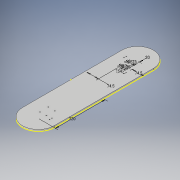
# Autodesk Inventor part: sfp_smartboard_lower_deck
Saved by Autodesk Inventor 2019 (Build 230136000, 136)
## iProperties
Created: 2019-02-09
Part Number: sfp_smartboard_lower_deck
Material: 一般
Document SubType Name: Modeling
Designer: drago
Density: 1 g/cm^3
Appearance: 既定
Author: drago
Autodesk Inventor part; units mm, degrees
ref_plane "YZ Plane" through (0, 0, 0) normal (1, 0, 0) x (0, 1, 0)
ref_plane "XZ Plane" through (0, 0, 0) normal (0, 1, 0) x (-1, 0, 0)
ref_plane "XY Plane" through (0, 0, 0) normal (0, 0, 1) x (1, 0, 0)
sketch "スケッチ1" plane through (0, 0, 0) normal (0, 1, 0) x (-1, 0, 0)
  point P0 (0, 0)
sketch "スケッチ2" plane through (0, 0, 0) normal (0, 1, 0) x (-1, 0, 0)
  line L0 (0.845, -60.969) -> (0.845, -330.969)
  line L1 (0, 0) -> (0, -1.5537)
  line L2 (-202.155, -60.969) -> (-202.155, -330.969)
  arc A0 (-202.155, -330.969) -> (0.845, -330.969) centre (-100.655, -330.969) ccw
  line L3 (0.845, -60.969) -> (0.845, 309.031)
  line L4 (-202.155, -60.969) -> (-202.155, 309.031)
  arc A1 (0.845, 309.031) -> (-202.155, 309.031) centre (-100.655, 309.031) ccw
  dimension "d0" = 270
  dimension "d1" = 203
  constraints: 10 end point, 4 point on circle, 3 vertical, 2 centre point, 2 tangent, 1 parallel
  measures "d0" distance of L0.start L0.end
  measures "d1" distance of L0.start L2.start
extrude "押し出し1" add sketch "スケッチ2" against normal blind 10
sketch "スケッチ4" plane through (0, -10, 0) normal (0, -1, 0) x (1, 0, 0)
  line L0 (73.655, -234.969) -> (127.655, -234.969)
  line L1 (127.655, -234.969) -> (127.655, -310.969)
  line L2 (127.655, -310.969) -> (73.655, -310.969)
  line L3 (73.655, -310.969) -> (73.655, -234.969)
  line L4 (202.155, -330.969) -> (202.155, 309.031) projected
  line L5 (-0.845, 309.031) -> (-0.845, -330.969) projected
  arc A0 (-0.845, -330.969) -> (202.155, -330.969) centre (100.655, -330.969) ccw projected
  line L6 (-0.845, -10.969) -> (202.155, -10.969)
  arc A1 (202.155, 309.031) -> (-0.845, 309.031) centre (100.655, 309.031) ccw projected
  line L7 (73.655, 213.031) -> (127.655, 213.031)
  line L8 (127.655, 213.031) -> (127.655, 289.031)
  line L9 (127.655, 289.031) -> (73.655, 289.031)
  line L10 (73.655, 289.031) -> (73.655, 213.031)
  circle A2 centre (79.655, -299.219) radius 2.75
  line L11 (100.655, -256.1001) -> (100.655, -272.969)
  circle A3 centre (79.655, -245.219) radius 2.75
  circle A4 centre (121.655, -299.219) radius 2.75
  circle A5 centre (121.655, -245.219) radius 2.75
  line L12 (73.655, 213.031) -> (127.655, 213.031)
  line L13 (127.655, 213.031) -> (127.655, 289.031)
  line L14 (127.655, 289.031) -> (73.655, 289.031)
  line L15 (73.655, 289.031) -> (73.655, 213.031)
  circle A6 centre (79.655, 277.281) radius 2.75
  line L16 (100.655, 234.1622) -> (100.655, 251.031)
  circle A7 centre (79.655, 223.281) radius 2.75
  circle A8 centre (121.655, 223.281) radius 2.75
  circle A9 centre (121.655, 277.281) radius 2.75
  point P0 (0, 0)
  dimension "d4" = 74.5
  dimension "d5" = 74.5
  dimension "d6" = 54
  dimension "d7" = 76
  dimension "d8" = 20
  dimension "d9" = 320
  dimension "d17" = 5.5
  dimension "d18" = 11.75
  dimension "d19" = 6
  dimension "d20" = 27
  dimension "d21" = 5.5
  dimension "d22" = 10.25
  dimension "d23" = 6
  constraints: 30 end point, 12 symmetric about line, 8 centre point, 2 midpoint, 2 parallel, 2 perpendicular, 1 horizontal, 1 vertical, 6 other
  measures "d4" distance between parallel lines of L4 L1
  measures "d5" distance between parallel lines of L5 L3
  measures "d6" distance of L0.start L0.end
  measures "d7" distance between parallel lines of L2 L0
  measures "d8" distance from line of A0.centre L2
  measures "d9" distance from line of A1.centre L6
  measures "d17" diameter of A2
  measures "d18" distance from line of L2 A2.centre
  measures "d19" distance from line of L3 A2.centre
  measures "d20" distance between parallel lines of L3 L11
  measures "d21" diameter of A3
  measures "d22" distance from line of L0 A3.centre
  measures "d23" distance from line of L3 A3.centre
hole "穴2" at (79.655, -10, -245.219) at (79.655, -10, -299.219) at (121.655, -10, -299.219) at (121.655, -10, -245.219) direction (0, 1, 0) diameter 5.5 end through all
hole "穴3" at (79.655, -10, 223.281) at (121.655, -10, 223.281) at (121.655, -10, 277.281) at (79.655, -10, 277.281) direction (0, 1, 0) diameter 5.5 end through all
sketch "スケッチ6" plane through (0, 0, 0) normal (0, 1, 0) x (1, 0, 0)
  circle A0 centre (153.655, -289.031) radius 6
  circle A1 centre (153.655, -274.031) radius 6
  line L0 (202.155, 330.969) -> (202.155, -309.031) projected
  arc A2 (-0.845, -309.031) -> (202.155, -309.031) centre (100.655, -309.031) ccw projected
  point P0 (0, 0)
  dimension "d40" = 12
  dimension "d41" = 12
  dimension "d42" = 15
  dimension "d43" = 48.5
  dimension "d44" = 48.5
  dimension "d45" = 20
  constraints: 2 centre point
  measures "d40" diameter of A0
  measures "d41" diameter of A1
  measures "d42" distance of A0.centre A1.centre
  measures "d43" distance from line of L0 A0.centre
  measures "d44" distance from line of L0 A1.centre
  measures "d45" vertical distance of A2.centre A0.centre
hole "穴4" at (153.655, 0, 274.031) at (153.655, 0, 289.031) direction (0, -1, 0) diameter 4.917 end through all thread size "M6x1" class "6H" standard "ANSI Metric M Profile"
sketch "スケッチ7" plane through (0, 0, 0) normal (0, 1, 0) x (1, 0, 0)
  circle A0 centre (47.655, 310.969) radius 6
  circle A1 centre (47.655, 295.969) radius 6
  arc A2 (202.155, 330.969) -> (-0.845, 330.969) centre (100.655, 330.969) ccw projected
  line L0 (-0.845, -309.031) -> (-0.845, 330.969) projected
  point P0 (0, 0)
  dimension "d53" = 12
  dimension "d54" = 12
  dimension "d55" = 15
  dimension "d56" = 20
  dimension "d57" = 48.5
  dimension "d58" = 48.5
  constraints: 2 centre point
  measures "d53" diameter of A0
  measures "d54" diameter of A1
  measures "d55" distance of A1.centre A0.centre
  measures "d56" vertical distance of A2.centre A0.centre
  measures "d57" distance from line of L0 A0.centre
  measures "d58" distance from line of L0 A1.centre
hole "穴5" at (47.655, 0, -310.969) at (47.655, 0, -295.969) direction (0, -1, 0) diameter 4.917 end through all thread size "M6x1" class "6H" standard "ANSI Metric M Profile"
